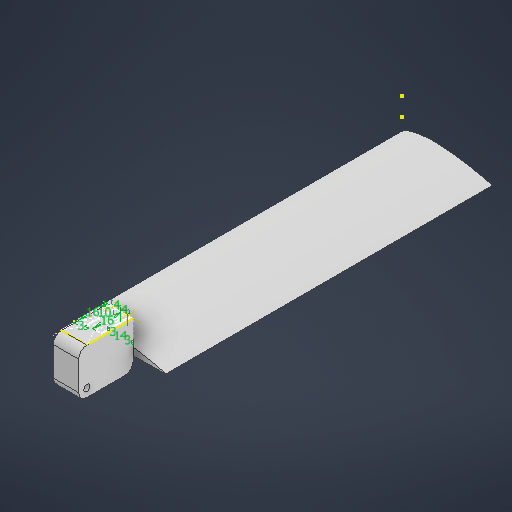
# Autodesk Inventor part: Pieza9
Saved by Autodesk Inventor 2026.1 (Build 301233000, 233)
## iProperties
Created: 2025-09-20
Part Number: Pieza9
Material: Genérico
Document SubType Name: Modeling
Designer: Usuario
Density: 1 g/cm^3
Appearance: Valor por defecto
Author: Usuario
Autodesk Inventor part; units mm, degrees
ref_plane "YZ Plane" through (0, 0, 0) normal (1, 0, 0) x (0, 1, 0)
ref_plane "XZ Plane" through (0, 0, 0) normal (0, 1, 0) x (-1, 0, 0)
ref_plane "XY Plane" through (0, 0, 0) normal (0, 0, 1) x (1, 0, 0)
sketch "Boceto7" plane through (0, 0, 0) normal (0, 0, 1) x (1, 0, 0)
  spline S0 degree 4 poles (50, -0.065) (47.6915, 0.7372) (46.9573, 0.8974) (40.7671, 2.3874) (35.0035, 3.3605) (30.032, 4.1261) (24.9861, 4.6118) (20.6928, 4.9661) (15.1988, 4.9352) (12.8969, 4.7695) (9.9976, 4.4267) (7.809, 4.0555) (5.1075, 3.3647) (3.8863, 2.9266) (2.647, 2.4985) (1.1391, 1.6236) (0.7673, 1.4533) (-0.5048, -0.0458) (0.7382, -0.8144) (1.1758, -0.9798) (2.6839, -1.3218) (3.9031, -1.3723) (5.1345, -1.4624) (7.8379, -1.4469) (10.0135, -1.3821) (12.9076, -1.2243) (15.2035, -1.1235) (20.686, -0.8568) (24.9753, -0.7094) (30.0115, -0.4903) (34.9865, -0.3186) (40.7206, -0.1592) (46.9254, -0.0826) (47.6748, -0.075) (50, -0.065) knots 0 0 0 0 0 0.079673 0.116564 0.156265 0.19586 0.235376 0.271963 0.30566 0.336519 0.364605 0.390772 0.415069 0.437588 0.456928 0.476371 0.494983 0.511973 0.530042 0.54789 0.566375 0.588202 0.612016 0.637863 0.665752 0.696534 0.730205 0.766764 0.806208 0.84565 0.885087 0.921634 1 1 1 1 1
  point P0 (0, 0)
  point P1 (47.5, 0.735)
  point P2 (45, 1.355)
  point P3 (40, 2.445)
  point P4 (35, 3.345)
  point P5 (30, 4.07)
  point P6 (25, 4.595)
  point P7 (20, 4.9)
  point P8 (15, 4.88)
  point P9 (12.5, 4.705)
  point P10 (10, 4.4)
  point P11 (7.5, 3.945)
  point P12 (5, 3.295)
  point P13 (3.75, 2.88)
  point P14 (2.5, 2.365)
  point P15 (1.25, 1.695)
  point P16 (0.625, 1.22)
  point P17 (0, 0)
  point P18 (0.625, -0.715)
  point P19 (1.25, -0.975)
  point P20 (2.5, -1.245)
  point P21 (3.75, -1.37)
  point P22 (5, -1.43)
  point P23 (7.5, -1.44)
  point P24 (10, -1.37)
  point P25 (12.5, -1.25)
  point P26 (15, -1.13)
  point P27 (20, -0.9)
  point P28 (25, -0.7)
  point P29 (30, -0.5)
  point P30 (35, -0.325)
  point P31 (40, -0.195)
  point P32 (45, -0.11)
  point P33 (47.5, -0.08)
  constraints: 35 other
extrude "Extrusión6" add sketch "Boceto7" along normal blind 180
sketch "Boceto8" plane through (0, 0, 180) normal (0, 0, 1) x (1, 0, 0)
  line L0 (0, 0) -> (50, 0) construction
  line L1 (0, -7.5) -> (50, -7.5)
  line L2 (50, -7.5) -> (50, 7.5)
  line L3 (50, 7.5) -> (0, 7.5)
  line L4 (0, 7.5) -> (0, -7.5)
  line L5 (0, -7.5) -> (50, 7.5) construction
  line L6 (50, -7.5) -> (0, 7.5) construction
  point P0 (25, 0)
  dimension "d23" = 50
  dimension "d24" = 15
  dimension "d25" = 50
  constraints: 14 end point, 3 midpoint, 2 horizontal, 2 parallel, 1 perpendicular, 1 other
  measures "d23" distance of L1.start L1.end
  measures "d24" distance between parallel lines of L1 L3
  measures "d25" distance of L0.start L0.end
extrude "Extrusión7" add sketch "Boceto8" along normal blind 30
sketch "Boceto9" plane through (0, 7.5, 180) normal (0, 1, 0) x (1, 0, 0)
  point P0 (0, 180)
sketch "Boceto10" plane through (0, 7.5, 180) normal (0, 1, 0) x (1, 0, 0)
  line L0 (50, 180) -> (50, 0) projected
  line L1 (0, -30) -> (50, -30) projected
  line L2 (50, 0) -> (0, 0)
  line L3 (0, 0) -> (0, -30)
  line L4 (0, -30) -> (50, -30)
  line L5 (50, -30) -> (50, 0)
  point P0 (0, 180)
  point P1 (50, -30)
  constraints: 8 end point, 2 parallel, 1 horizontal, 1 perpendicular
extrude "Extrusión8" add sketch "Boceto10" along normal blind 10
sketch "Boceto11" plane through (50, -7.5, 180) normal (1, 0, 0) x (0, 0, -1)
  line L0 (0, 25) -> (-30, 25) construction
  line L1 (0, 0) -> (-30, 0) construction
  line L2 (-30, 25) -> (0, 25) construction
  line L3 (0, 25) -> (0, 0) construction
  line L4 (0, 0) -> (-30, 0) construction
  line L5 (-30, 0) -> (-30, 25) construction
  circle A0 centre (-25.5, 4.5) radius 4.5 construction
  line L6 (-30, 0) -> (-30, 25) projected
  circle A1 centre (-25.5, 4.5) radius 1.75
  point P0 (180, 7.5)
  dimension "d30" = 9
  dimension "d31" = 3.5
  constraints: 8 end point, 2 centre point, 2 parallel, 2 tangent, 1 coincident, 1 horizontal, 1 perpendicular
  measures "d30" diameter of A0
  measures "d31" diameter of A1
extrude "Extrusión9" cut sketch "Boceto11" against normal up to next
fillet "Empalme2" radius 4.5 1 edges at (25, -7.5, 210)
sketch "Boceto12" plane through (0, -7.5, 180) normal (0, -1, 0) x (1, 0, 0)
  line L0 (50, 30) -> (0, 30) construction
  line L1 (50, -180) -> (50, 0) projected
  line L2 (0, 30) -> (50, 30) construction
  line L3 (50, 30) -> (50, 0) construction
  line L4 (50, 0) -> (0, 0) construction
  line L5 (0, 0) -> (0, 30) construction
  line L6 (0, 30) -> (18, 30)
  line L7 (18, 30) -> (18, 0)
  line L8 (18, 0) -> (0, 0)
  line L9 (0, 0) -> (0, 30)
  line L10 (50, 30) -> (32, 30)
  line L11 (32, 30) -> (32, 0)
  line L12 (32, 0) -> (50, 0)
  line L13 (50, 0) -> (50, 30)
  point P0 (0, -180)
  point P1 (32, 15)
  point P2 (18, 15)
  dimension "d35" = 14
  dimension "d36" = 18
  constraints: 24 end point, 6 parallel, 3 horizontal, 3 perpendicular, 2 midpoint, 2 point on line
  measures "d35" distance of point (32, 15) point (18, 15)
  measures "d36" distance between parallel lines of L7 L5
extrude "Extrusión10" cut sketch "Boceto12" against normal up to next
sketch "Boceto13" plane through (0, 17.5, 180) normal (0, 1, 0) x (1, 0, 0)
  point P0 (0, 180)
fillet "Empalme3" radius 4.5 1 edges at (25, 17.5, 210)
fillet "Empalme4" radius 4.5 1 edges at (25, -7.5, 180)
sketch "Boceto14" plane through (0, 0, 180) normal (0, 0, -1) x (-1, 0, 0)
  line L0 (-32, 17.5) -> (-18, 17.5) construction
  line L1 (-18, 17.5) -> (-18, 7.5) construction
  line L2 (-18, 7.5) -> (-32, 7.5) construction
  line L3 (-32, 7.5) -> (-32, 17.5) construction
  line L4 (-30.5, 17.5) -> (-27.5, 17.5)
  line L5 (-27.5, 17.5) -> (-27.5, 7.5)
  line L6 (-27.5, 7.5) -> (-30.5, 7.5)
  line L7 (-30.5, 7.5) -> (-30.5, 17.5)
  line L8 (-32, 17.5) -> (-18, 7.5) construction
  line L9 (-32, 7.5) -> (-18, 17.5) construction
  line L10 (-30.5, 17.5) -> (-27.5, 7.5) construction
  line L11 (-30.5, 7.5) -> (-27.5, 17.5) construction
  line L12 (-22.5, 17.5) -> (-19.5, 17.5)
  line L13 (-19.5, 17.5) -> (-19.5, 7.5)
  line L14 (-19.5, 7.5) -> (-22.5, 7.5)
  line L15 (-22.5, 7.5) -> (-22.5, 17.5)
  line L16 (-22.5, 17.5) -> (-19.5, 7.5) construction
  line L17 (-22.5, 7.5) -> (-19.5, 17.5) construction
  point P0 (0, 0)
  point P1 (-25, 12.5)
  point P2 (-29, 12.5)
  point P3 (-21, 12.5)
  point P4 (-25, 12.5)
  dimension "d41" = 14
  dimension "d42" = 10
  dimension "d43" = 3
  dimension "d44" = 4
  dimension "d45" = 3
  dimension "d46" = 4
  constraints: 36 end point, 6 parallel, 4 midpoint, 4 point on line, 3 horizontal, 3 perpendicular
  measures "d41" distance of L1.end L2.end
  measures "d42" distance of L0.end L1.end
  measures "d43" distance of L5.end L6.end
  measures "d44" distance of point (-25, 12.5) point (-29, 12.5)
  measures "d45" distance of L13.end L14.end
  measures "d46" distance of point (-21, 12.5) point (-25, 12.5)
sketch "Boceto15" plane through (0, 17.5, 180) normal (0, 1, 0) x (1, 0, 0)
  line L0 (32, -25.5) -> (32, 0) projected
  line L1 (18, -25.5) -> (32, -25.5) projected
  line L2 (32, 0) -> (18, 0)
  line L3 (18, 0) -> (18, -25.5)
  line L4 (18, -25.5) -> (32, -25.5)
  line L5 (32, -25.5) -> (32, 0)
  line L6 (30.5, 0) -> (27.5, 0)
  line L7 (27.5, 0) -> (27.5, -16)
  line L8 (27.5, -16) -> (30.5, -16)
  line L9 (30.5, -16) -> (30.5, 0)
  line L10 (22.5, 0) -> (19.5, 0)
  line L11 (19.5, 0) -> (19.5, -16)
  line L12 (19.5, -16) -> (22.5, -16)
  line L13 (22.5, -16) -> (22.5, 0)
  line L14 (30.5, 0) -> (27.5, -16) construction
  line L15 (19.5, 0) -> (22.5, -16) construction
  line L16 (22.5, 0) -> (19.5, -16) construction
  line L17 (27.5, 0) -> (30.5, -16) construction
  line L18 (18, -30) -> (18, -25.5) construction
  line L19 (32, 0) -> (18, -25.5) construction
  line L20 (32, 0) -> (18, 0) construction
  line L21 (18, 0) -> (32, -25.5) construction
  point P0 (0, 180)
  point P1 (30.5, 0)
  point P2 (27.5, 0)
  point P3 (29, 0)
  point P4 (21, 0)
  dimension "d47" = 16
  dimension "d48" = 3
  dimension "d49" = 16
  constraints: 34 end point, 7 parallel, 3 horizontal, 2 perpendicular, 1 point on line, 1 vertical, 5 other
  measures "d47" distance of L7.end L6.end
  measures "d48" distance of L12.end L11.end
  measures "d49" distance of L11.end L10.end
